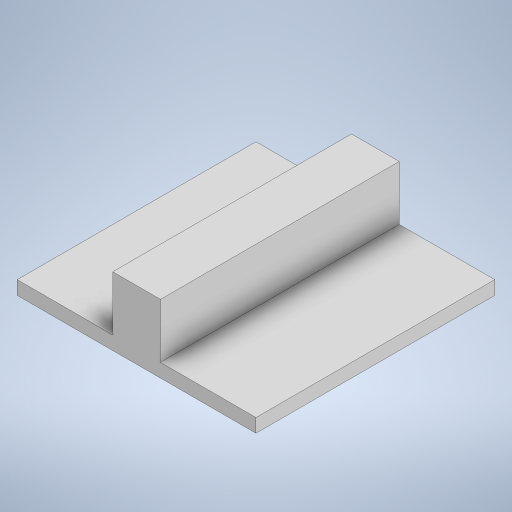
# Autodesk Inventor part: ZadBabkaOsnova
Saved by Autodesk Inventor 2024 (Build 280153000, 153)
## iProperties
Created: 2023-08-28
Part Number: ZadBabkaOsnova
Material: Generic
Document SubType Name: Modeling
Designer: KirikDK
Density: 1 g/cm^3
Appearance: Default
Author: KirikDK
Autodesk Inventor part; units mm, degrees
ref_plane "YZ Plane" through (0, 0, 0) normal (1, 0, 0) x (0, 1, 0)
ref_plane "XZ Plane" through (0, 0, 0) normal (0, 1, 0) x (-1, 0, 0)
ref_plane "XY Plane" through (0, 0, 0) normal (0, 0, 1) x (1, 0, 0)
sketch "Sketch1" plane through (0, 0, 0) normal (0, 1, 0) x (-1, 0, 0)
  line L0 (50, 50) -> (-125, 50)
  line L1 (-125, 50) -> (-125, -125)
  line L2 (-125, -125) -> (50, -125)
  line L3 (50, -125) -> (50, 50)
  point P0 (0, 0)
  dimension "d0" = 175
  dimension "d1" = 175
  constraints: 8 end point, 2 parallel, 1 horizontal, 1 perpendicular
  measures "d0" distance of L2.end L0.start
  measures "d1" distance of L0.start L0.end
extrude "Extrusion1" add sketch "Sketch1" along normal blind 10
sketch "Sketch2" plane through (0, 10, 0) normal (0, 1, 0) x (1, 0, 0)
  line L0 (-50, -50) -> (125, -50) projected
  line L1 (20, -50) -> (55, -50)
  line L2 (55, -50) -> (55, 125)
  line L3 (55, 125) -> (20, 125)
  line L4 (20, 125) -> (20, -50)
  line L5 (-50, 125) -> (-50, -50) projected
  line L6 (125, -50) -> (125, 125) projected
  point P0 (0, 0)
  dimension "d4" = 70
  dimension "d5" = 70
  constraints: 8 end point, 2 parallel, 1 horizontal, 1 perpendicular, 1 point on line
  measures "d4" distance between parallel lines of L5 L4
  measures "d5" distance between parallel lines of L2 L6
extrude "Extrusion2" add sketch "Sketch2" along normal blind 40
body "Solid1"
